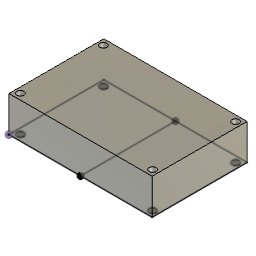
magp_base_plate (Autodesk Fusion 360 archive; units mm, degrees)
design "power_supply_base"
Autodesk Fusion 360 part; units mm, degrees
sketch "スケッチ1" plane through (0, 0, 0) normal (0, 0, 1) x (1, 0, 0)
  line L0 (0, 0) -> (72.4, 0)
  line L1 (72.4, 0) -> (72.4, 48)
  line L2 (72.4, 48) -> (0, 48)
  line L3 (0, 48) -> (0, 0)
  circle A0 centre (2.8, 45) radius 1.75
  circle A1 centre (69.6, 45) radius 1.75
  circle A2 centre (69.6, 3) radius 1.75
  circle A3 centre (2.8, 3) radius 1.75
  line L4 (36.2, 48) -> (36.2, 0)
  point P0 (36.2, 48)
  point P1 (36.2, 0)
  dimension "d1" = 72.4
  dimension "d2" = 48
  dimension "d3" = 3.5
  dimension "d7" = 3
  dimension "d8" = 2.8
  dimension "d9" = 2.8
  dimension "d10" = 3
  dimension "d11" = 2.8
  dimension "d12" = 3
  dimension "d13" = 3
  dimension "d14" = 2.8
  constraint horizontal L0
  constraint vertical L1
  constraint horizontal L2
  constraint vertical L3
  constraint coincident L0.start L3.end
  constraint midpoint L2 P0
  constraint midpoint L0 P1
  constraint coincident P0 L4.start
  constraint coincident P1 L4.end
  constraint equal A0 A1
  constraint equal A0 A2
  constraint equal A0 A3
  measures "d1" distance of L0.start L0.end
  measures "d2" distance of L0.start L2.end
  measures "d3" diameter of A0
  measures "d7" distance of L2 A0.centre
  measures "d8" distance of L3 A0.centre
  measures "d9" distance of L1 A1.centre
  measures "d10" distance of L2 A1.centre
  measures "d11" distance of L3 A3.centre
  measures "d12" distance of L0 A3.centre
  measures "d13" distance of L0 A2.centre
  measures "d14" distance of L1 A2.centre
extrude "押し出し1" add sketch "スケッチ1" along normal blind 18 contours L0 L2 L3 L4 | L0 L1 L2 L4 | A0 | A1 | A2 | A3
extrude "押し出し2" cut sketch "スケッチ1" along normal blind 18 contours A0 | A1 | A2 | A3

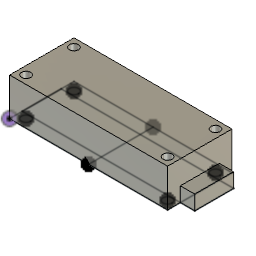
design "motor_driver"
Autodesk Fusion 360 part; units mm, degrees
sketch "スケッチ1" plane through (0, 0, 0) normal (0, 0, 1) x (1, 0, 0)
  line L0 (0, 0) -> (62.5, 0)
  line L1 (62.5, 0) -> (62.5, 25.5)
  line L2 (62.5, 25.5) -> (0, 25.5)
  line L3 (0, 25.5) -> (0, 0)
  circle A0 centre (3.275, 22.225) radius 1.775
  circle A1 centre (3.275, 3.275) radius 1.775
  circle A2 centre (59.225, 22.225) radius 1.775
  circle A3 centre (59.225, 3.275) radius 1.775
  line L4 (0, 20.45) -> (68.2, 20.45)
  line L5 (68.2, 20.45) -> (68.2, 5.05)
  line L6 (68.2, 5.05) -> (0, 5.05)
  line L7 (0, 5.05) -> (0, 20.45)
  line L8 (31.25, 25.5) -> (31.25, 0)
  point P0 (3.275, 22.225)
  point P1 (3.275, 3.275)
  point P2 (59.225, 3.275)
  point P3 (59.225, 22.225)
  point P4 (31.25, 25.5)
  point P5 (31.25, 0)
  dimension "d1" = 62.5
  dimension "d2" = 25.5
  dimension "d3" = 3.275
  dimension "d4" = 3.275
  dimension "d5" = 3.55
  dimension "d6" = 3.275
  dimension "d7" = 3.275
  dimension "d9" = 3.275
  dimension "d10" = 3.275
  dimension "d11" = 3.275
  dimension "d12" = 3.275
  dimension "d15" = 68.2
  constraint horizontal L0
  constraint vertical L1
  constraint horizontal L2
  constraint vertical L3
  constraint coincident L0.start L3.end
  constraint coincident P0 A0.centre
  constraint coincident P1 A1.centre
  constraint coincident P3 A2.centre
  constraint coincident P2 A3.centre
  constraint horizontal L4
  constraint vertical L5
  constraint horizontal L6
  constraint vertical L7
  constraint coincident L3 L4.start
  constraint tangent A2 L4
  constraint tangent A3 L6
  constraint equal A0 A2
  constraint equal A0 A1
  constraint equal A0 A3
  constraint coincident L2 P4
  constraint midpoint L2 P4
  constraint midpoint L0 P5
  constraint coincident P4 L8.start
  constraint coincident P5 L8.end
  measures "d1" distance of L0.start L0.end
  measures "d2" distance of L0.start L2.end
  measures "d3" distance of L2 P0
  measures "d4" distance of L3 P0
  measures "d5" diameter of A0
  measures "d6" distance of L3 P1
  measures "d7" distance of L0 P1
  measures "d9" distance of L0 P2
  measures "d10" distance of L1 P2
  measures "d11" distance of L1 P3
  measures "d12" distance of L2 P3
  measures "d15" distance of L4.start L4.end
extrude "押し出し1" add sketch "スケッチ1" along normal blind 15 contours L0 L3 L6 L8 | L0 L1 L6 L8 | L3 L4 L6 L7 L8 | L1 L4 L6 L8 | L2 L3 L4 L8 | L1 L2 L4 L8
extrude "押し出し2" add sketch "スケッチ1" along normal blind 5.75 contours L1 L4 L5 L6
equation "d3 = 1.7 mm + ( ( 3.15 / 2 ) * 1 mm )"
equation "d5 = 3.15 mm + 0.4 mm"

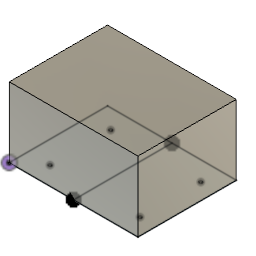
design "jetson_orin_case"
Autodesk Fusion 360 part; units mm, degrees
sketch "スケッチ1" plane through (0, 0, 0) normal (0, 0, 1) x (1, 0, 0)
  line L0 (0, 0) -> (123, 0)
  line L1 (123, 0) -> (123, 94)
  line L2 (123, 94) -> (0, 94)
  line L3 (0, 94) -> (0, 0)
  circle A0 centre (21.5, 17.5) radius 1.25
  circle A1 centre (21.5, 75.5) radius 1.25
  circle A2 centre (107.5, 17.5) radius 1.25
  circle A3 centre (107.5, 75.5) radius 1.25
  line L4 (61.5, 0) -> (61.5, 94)
  point P0 (61.5, 0)
  point P1 (61.5, 94)
  dimension "d1" = 123
  dimension "d2" = 94
  dimension "d5" = 21.5
  dimension "d6" = 17.5
  dimension "d7" = 2.5
  dimension "d10" = 18.5
  dimension "d11" = 21.5
  dimension "d12" = 18.5
  dimension "d13" = 15.5
  dimension "d14" = 15.5
  dimension "d15" = 17.5
  constraint horizontal L0
  constraint vertical L1
  constraint horizontal L2
  constraint vertical L3
  constraint coincident L0.start L3.end
  constraint midpoint L0 P0
  constraint midpoint L2 P1
  constraint coincident P0 L4.start
  constraint coincident P1 L4.end
  constraint equal A1 A3
  constraint equal A1 A2
  constraint equal A0 A1
  measures "d1" distance of L0.start L0.end
  measures "d2" distance of L0.start L2.end
  measures "d5" distance of L3 A0.centre
  measures "d6" distance of L0 A0.centre
  measures "d7" diameter of A1
  measures "d10" distance of L2 A1.centre
  measures "d11" distance of L3 A1.centre
  measures "d12" distance of L2 A3.centre
  measures "d13" distance of L1 A3.centre
  measures "d14" distance of L1 A2.centre
  measures "d15" distance of L0 A2.centre
extrude "押し出し1" add sketch "スケッチ1" along normal blind 67 contours L0 L2 L3 L4 | L0 L1 L2 L4 | A0 | A1 | A2 | A3
extrude "押し出し2" cut sketch "スケッチ1" along normal blind 15 contours A0 | A1 | A2 | A3
sketch "スケッチ2" plane through (0, 94, 0) normal (0, -1, 0) x (1, 0, 0)
  line L0 (0, 0) -> (123, 0)
  line L1 (123, 0) -> (123, 67)
  line L2 (123, 67) -> (0, 67)
  line L3 (0, 67) -> (0, 0)
  circle A0 centre (36.9, 49.6) radius 3.1
  circle A1 centre (86.1, 49.6) radius 3.1
  line L4 (123, 0) -> (0, 0)
  line L5 (0, 0) -> (0, 67)
  line L6 (0, 67) -> (123, 67)
  line L7 (123, 67) -> (123, 0)
  dimension "d20" = 6.2
  dimension "d21" = 6.2
  dimension "d22" = 36.9
  dimension "d23" = 36.9
  dimension "d24" = 17.4
  dimension "d25" = 17.4
  measures "d20" diameter of A0
  measures "d21" diameter of A1
  measures "d22" distance of L3 A0.centre
  measures "d23" distance of L1 A1.centre
  measures "d24" distance of L2 A1.centre
  measures "d25" distance of L2 A0.centre
extrude "押し出し3" add sketch "スケッチ2" along normal blind 0 and the other way blind 10 contours A0 | A1
